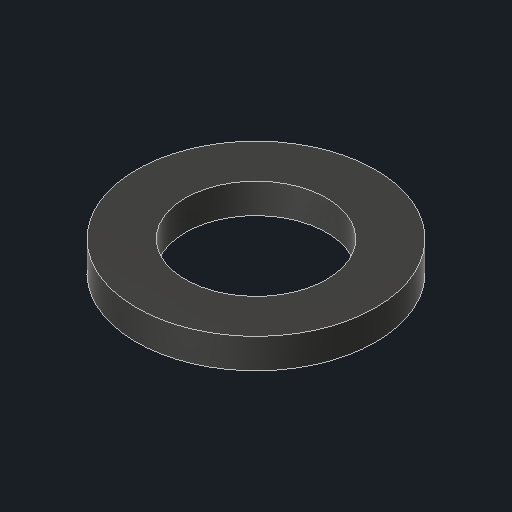
# Autodesk Inventor part: 217-6937
Saved by Autodesk Inventor 2023 (Build 270158000, 158)
## iProperties
Created: 2020-11-14
Part Number: 217-6937
Material: Acetal Resin, Black
Document SubType Name: Modeling
Density: 1.425 g/cm^3
Appearance: Smooth - Black
Mass: 312.75 g
Surface Area: 212.817 cm^2
Volume: 115.833 cm^3
Revision Number: 0
Autodesk Inventor part; units mm, degrees
ref_plane "YZ Plane" through (0, 0, 0) normal (1, 0, 0) x (0, 1, 0)
ref_plane "XZ Plane" through (0, 0, 0) normal (0, 1, 0) x (-1, 0, 0)
ref_plane "XY Plane" through (0, 0, 0) normal (0, 0, 1) x (1, 0, 0)
sketch "Sketch1" plane through (0, 0, 0) normal (0, 0, 1) x (1, 0, 0)
  line L0 (3.75, 0.7937) -> (3.75, -0.7937)
  line L1 (3.75, -0.7937) -> (6.35, -0.7937)
  line L2 (6.35, -0.7937) -> (6.35, 0.7937)
  line L3 (6.35, 0.7937) -> (3.75, 0.7937)
  line L4 (0, 0) -> (0, 3.8331) construction
  line L5 (0, 0) -> (3.75, 0.7937) construction
  line L6 (0, 0) -> (3.75, -0.7937) construction
  point P0 (0, 0)
  dimension "d13" = 7.5
  dimension "d14" = 12.7
  dimension "d15" = 1.5875
  constraints: 14 end point, 3 equal length, 2 perpendicular, 2 vertical, 1 coincident, 1 horizontal
  measures "d13" diameter of L0 L4
  measures "d14" diameter of L2 L4
  measures "d15" distance between parallel lines of L1 L3
revolve "Revolution1" add sketch "Sketch1" angle 360 about axis through (0, 0, 0) along (0, 1, 0)
thread "Thread2" size "10-32 UNF" class "2B" standard "ANSI Unified Screw Threads" length 9.525
thread "Thread1" size "10-32 UNF" class "2B" standard "ANSI Unified Screw Threads" length 9.525
sketch "Sketch2" plane through (0, 0.7937, 12.7) normal (0, 1, 0) x (1, 0, 0)
  line L0 (-7.3323, 12.7) -> (-3.6662, 19.05)
  line L1 (-3.6662, 19.05) -> (3.6662, 19.05)
  line L2 (3.6662, 19.05) -> (7.3323, 12.7)
  line L3 (7.3323, 12.7) -> (3.6662, 6.35)
  line L4 (3.6662, 6.35) -> (-3.6662, 6.35)
  line L5 (-3.6662, 6.35) -> (-7.3323, 12.7)
  circle A0 centre (0, 12.7) radius 6.35 projected
  point P0 (-5.4993, 9.525)
  point P1 (-5.4993, 15.875)
  point P2 (0, 19.05)
  point P3 (5.4993, 15.875)
  point P4 (5.4993, 9.525)
  point P5 (0, 6.35)
  constraints: 12 end point, 1 coincident, 1 horizontal, 1 tangent, 13 other
extrude "OD Hex" [suppressed]
sketch "Sketch3" plane through (0, 14.2875, 12.7) normal (0, 1, 0) x (1, 0, 0)
  circle A0 centre (0, 12.7) radius 4.7625
  circle A1 centre (0, 12.7) radius 76.2
  point P0 (0, 12.7)
  dimension "d8" = 152.4
  dimension "d17" = 12.7
  constraints: 2 centre point, 1 coincident, 1 concentric
  measures "d8" diameter of A1
extrude "Hex Round" [suppressed]
mirror "Mirror1" [suppressed]
sketch "Sketch4" plane through (0, 0.7937, 12.7) normal (0, 1, 0) x (1, 0, 0)
  circle A0 centre (0, 12.7) radius 3.75 projected
  line L0 (-4.3301, 12.7) -> (-2.1651, 16.45)
  line L1 (-2.1651, 16.45) -> (2.1651, 16.45)
  line L2 (2.1651, 16.45) -> (4.3301, 12.7)
  line L3 (4.3301, 12.7) -> (2.1651, 8.95)
  line L4 (2.1651, 8.95) -> (-2.1651, 8.95)
  line L5 (-2.1651, 8.95) -> (-4.3301, 12.7)
  constraints: 12 end point, 1 coincident, 1 horizontal, 1 tangent, 13 other
extrude "ID Hex" [suppressed]
equation "\"d13\" = ID"
equation "\"d14\" = OD"
equation "\"d15\" = Length"
equation "\"d27\" = d25"
equation "\"d17\" = OD"
equation "\"ID\" = 7.5"
equation "\"OD\" = 12.7"
equation "\"Length\" = 1.5875"
equation "\"d25\" = 9.525"
body "Solid114"
body "Solid1"
